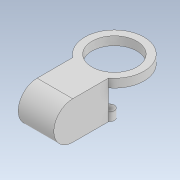
# Autodesk Inventor part: left_thigh
Saved by Autodesk Inventor 2020 (Build 240168000, 168)
## iProperties
Created: 2021-01-12
Part Number: left_thigh
Material: Generic
Document SubType Name: Modeling
Designer: DELL
Density: 1 g/cm^3
Appearance: Default
Author: DELL
Autodesk Inventor part; units mm, degrees
ref_plane "YZ Plane" through (0, 0, 0) normal (1, 0, 0) x (0, 1, 0)
sketch "Sketch2" plane through (0, 0, 0) normal (0, 1, 0) x (-1, 0, 0)
  circle A0 centre (-25, -83.5) radius 36 construction
  line L0 (-25, -83.5) -> (-61, -83.5) construction
  line L1 (-25, -83.5) -> (4.6941, -63.1466) construction
  circle A1 centre (-25, -83.5) radius 41.5
  circle A2 centre (-25, -83.5) radius 28
  arc A3 (-8.1325, -61.1508) -> (0, -50.3752) centre (-4.0663, -55.763) ccw
  arc A4 (-50, -50.3752) -> (-39.3017, -57.0193) centre (-45.9337, -55.763) ccw
  line L2 (-25, -83.5) -> (-4.0663, -55.763) construction
  circle A5 centre (-25, -83.5) radius 31.5
  line L3 (0, -50.3752) -> (0, 0)
  line L4 (-50, -50.3752) -> (-50, 0)
  line L5 (0, 0) -> (-50, 0)
  line L6 (-25, 0) -> (-25, -83.5) construction
  point P0 (15.9829, -76.969)
  point P1 (13.8342, -68.866)
  point P2 (-39.2078, -55.1936)
  point P3 (-41.8675, -61.1508)
  point P4 (-8.1325, -61.1508)
  dimension "d1" = 72
  dimension "d5" = 83
  dimension "d6" = 56
  dimension "d7" = 63
  dimension "d11" = 50
  dimension "d31" = 83.5
  constraints: 15 end point, 11 point on circle, 6 centre point, 4 coincident, 4 tangent, 3 vertical, 1 horizontal, 1 midpoint, 1 point on line
  measures "d1" diameter of A0
  measures "d5" diameter of A1
  measures "d6" diameter of A2
  measures "d7" diameter of A5
  measures "d11" distance of L3.end L4.end
  measures "d31" distance from line of L5 A1.centre
ref_plane "Work Plane1" through (0, -14.5, 0) normal (0, 1, 0) x (-1, 0, 0)
ref_plane "Work Plane2" through (0, 14.5, 0) normal (0, 1, 0) x (-1, 0, 0)
extrude "Extrusion1" add sketch "Sketch2" along normal blind 12 from surface at 14.5 contours A1 A4 A5 A3 | A3 A5 A4 A1
extrude "Extrusion2" add sketch "Sketch2" against normal blind 12 from surface at -14.5 contours A3 A5 A4 A1 | A3 A2 A4 A5 picked at (-44.9519, -51.1635) picked at (-38.3765, -56.444)
extrude "Extrusion3" add sketch "Sketch2" along normal mid plane 53 contours A1 L4 L5 L3
sketch "Sketch3" plane through (0, 0, 0) normal (1, 0, 0) x (0, 1, 0)
  line L0 (26.5, 0) -> (-26.5, 0) projected
  circle A0 centre (0, 0) radius 26.5
  constraints: 1 coincident, 1 horizontal alignment, 2 other
extrude "Extrusion4" add sketch "Sketch3" along normal up to surface (50 mm away)
body "Solid1"
